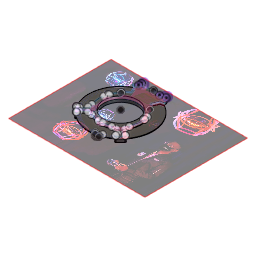
2023_02_18_DroneSoccerGoalFormat v3 (Autodesk Fusion 360 design; units mm, degrees)
Autodesk Fusion 360 part; units mm, degrees
note: some values were not read from the file. Set by a fixed rule: which face or edge a step refers to.
sketch "Sketch1" plane through (0, 0, 0) normal (0, 0, 1) x (1, 0, 0)
  circle A0 centre (0, 0) radius 30
  dimension "d1" = 60
  constraint coincident A0.centre origin
  measures "d1" diameter of A0
sketch "Sketch2" plane through (0, 0, 0) normal (0, 0, 1) x (1, 0, 0)
  line L0 (0.0532, -39.3057) -> (0.0532, -31.0517)
  line L1 (0.0532, -31.0517) -> (5.2469, -34.1533)
  line L2 (5.9386, -36.8958) -> (5.0815, -38.3311)
  line L3 (3.3644, -39.3057) -> (0.0532, -39.3057)
  line L4 (0.0532, -39.3057) -> (-3.258, -39.3057)
  line L5 (0.0532, -31.0517) -> (-5.1405, -34.1533)
  line L6 (-5.8322, -36.8958) -> (-4.9751, -38.3311)
  line L7 (-6.8576, -35.1787) -> (0.0532, -35.1787)
  line L8 (6.964, -35.1787) -> (0.0532, -35.1787)
  line L9 (0, 0) -> (-47, -35)
  line L10 (-47, -35) -> (-50.3407, -30.5139)
  line L11 (-50.6925, -28.9018) -> (-50.6943, -28.91)
  line L12 (-48.4045, -27.4507) -> (-45.0572, -29.2075)
  line L13 (-43.9952, -29.1241) -> (-35.2985, -22.6478)
  line L14 (-34.5132, -19.6138) -> (-37.2797, -13.4877)
  line L15 (-37.2164, -12.5462) -> (-35.0998, -9.1596)
  line L16 (-34.5983, -8.6155) -> (-32.5036, -7.0556)
  line L17 (-32.5036, -7.0556) -> (-24.2886, -18.0872)
  line L18 (0, 0) -> (0, 59)
  spline S0 degree 5 poles (0, 59) (-0.1827, 59.02) (-0.5488, 59.0563) (-1.1, 59.0994) (-1.8389, 59.134) (-2.7694, 59.1396) (-3.7076, 59.1081) (-4.6547, 59.0407) (-5.613, 58.9396) (-6.5861, 58.8081) (-7.5782, 58.6505) (-8.5938, 58.4709) (-9.637, 58.2733) (-10.7108, 58.0605) (-11.8165, 57.8337) (-12.953, 57.5917) (-14.1166, 57.3315) (-15.3013, 57.0494) (-16.4983, 56.7421) (-17.6962, 56.4075) (-18.8812, 56.0461) (-20.0369, 55.6616) (-21.1435, 55.2619) (-22.1835, 54.8583) (-23.1442, 54.4622) (-24.0258, 54.085) (-24.8384, 53.7327) (-25.6255, 53.4115) (-26.4188, 53.1074) (-27.16, 52.7706) (-27.7715, 52.3532) (-28.1746, 51.8252) (-28.3371, 51.2074) (-28.2837, 50.5744) (-28.0598, 50.0112) (-27.7047, 49.5822) (-27.218, 49.2903) (-26.5845, 49.0991) (-25.8011, 48.9581) (-24.9091, 48.8302) (-24.0064, 48.7073) (-23.2054, 48.5909) (-22.5994, 48.4787) (-22.2292, 48.3506) (-22.0395, 48.15) (-21.9198, 47.807) (-21.7816, 47.2816) (-21.5743, 46.5694) (-21.274, 45.6894) (-20.8803, 44.677) (-20.4088, 43.5748) (-19.8868, 42.4257) (-19.3496, 41.2728) (-18.8364, 40.1572) (-18.3867, 39.1164) (-18.0364, 38.183) (-17.8142, 37.3825) (-17.737, 36.733) (-17.8129, 36.2378) (-18.0462, 35.8787) (-18.443, 35.6058) (-19.0127, 35.3379) (-19.7561, 34.9915) (-20.657, 34.5019) (-21.6709, 33.8519) (-22.7199, 33.0863) (-23.7129, 32.2831) (-24.561, 31.5304) (-25.1962, 30.9002) (-25.5866, 30.4256) (-25.7572, 30.0716) (-25.7979, 29.7223) (-25.8113, 29.2507) (-25.8549, 28.5945) (-25.9293, 27.7723) (-26.0025, 26.8503) (-26.0238, 25.9241) (-25.9422, 25.0938) (-25.722, 24.4425) (-25.3404, 24.0341) (-24.7859, 23.9095) (-24.0562, 24.0833) (-23.1567, 24.5434) (-22.0989, 25.2573) (-20.899, 26.1767) (-19.5762, 27.2425) (-18.1514, 28.3898) (-16.6454, 29.5532) (-15.078, 30.6708) (-13.4656, 31.6909) (-11.8213, 32.5724) (-10.1553, 33.2835) (-8.4753, 33.8004) (-6.7868, 34.1063) (-5.0934, 34.19) (-3.3972, 34.045) (-2.0389, 33.7434) (-1.0197, 33.4125) (-0.3399, 33.1452) (0, 33) knots 0 0 0 0 0 0 0.01052632 0.02105263 0.03157895 0.04210526 0.05263158 0.06315789 0.07368421 0.08421053 0.09473684 0.10526316 0.11578947 0.12631579 0.13684211 0.14736842 0.15789474 0.16842105 0.17894737 0.18947368 0.2 0.21052632 0.22105263 0.23157895 0.24210526 0.25263158 0.26315789 0.27368421 0.28421053 0.29473684 0.30526316 0.31578947 0.32631579 0.33684211 0.34736842 0.35789474 0.36842105 0.37894737 0.38947368 0.4 0.41052632 0.42105263 0.43157895 0.44210526 0.45263158 0.46315789 0.47368421 0.48421053 0.49473684 0.50526316 0.51578947 0.52631579 0.53684211 0.54736842 0.55789474 0.56842105 0.57894737 0.58947368 0.6 0.61052632 0.62105263 0.63157895 0.64210526 0.65263158 0.66315789 0.67368421 0.68421053 0.69473684 0.70526316 0.71578947 0.72631579 0.73684211 0.74736842 0.75789474 0.76842105 0.77894737 0.78947368 0.8 0.81052632 0.82105263 0.83157895 0.84210526 0.85263158 0.86315789 0.87368421 0.88421053 0.89473684 0.90526316 0.91578947 0.92631579 0.93684211 0.94736842 0.95789474 0.96842105 0.97894737 0.98947368 1 1 1 1 1 1
  line L19 (-18.95, 56.1909) -> (-30.95, 51.1909)
  line L20 (-22.4748, 54.735) -> (-22.2313, 59.7077)
  line L21 (-21.5993, 60.1653) -> (-20.6365, 59.9004)
  line L22 (-20.1056, 61.8303) -> (-21.1577, 62.1197)
  arc A0 (-21.5993, 60.1653) -> (-22.2313, 59.7077) centre (-21.7319, 59.6832) ccw
  arc A1 (-21.3482, 62.5395) -> (-21.1577, 62.1197) centre (-21.0781, 62.409) ccw
  arc A2 (-20.6365, 59.9004) -> (-20.1056, 61.8303) centre (-18.7963, 60.4321) ccw
  spline S1 degree 5 poles (-21.3482, 62.5395) (-21.2588, 62.6491) (-21.0782, 62.8581) (-20.8015, 63.1417) (-20.4212, 63.4598) (-19.9273, 63.7557) (-19.4168, 63.9482) (-18.8942, 64.0357) (-18.3672, 64.0174) (-17.8475, 63.894) (-17.3471, 63.6688) (-16.8752, 63.348) (-16.4352, 62.9422) (-16.0208, 62.4678) (-15.6183, 61.9452) (-15.2114, 61.3961) (-14.786, 60.8402) (-14.334, 60.2934) (-13.8593, 59.7639) (-13.3785, 59.2517) (-12.9142, 58.7523) (-12.5748, 58.3573) (-12.3465, 58.0607) (-12.2072, 57.8625) (-12.1407, 57.7633) knots 0 0 0 0 0 0 0.05 0.1 0.15 0.2 0.25 0.3 0.35 0.4 0.45 0.5 0.55 0.6 0.65 0.7 0.75 0.8 0.85 0.9 0.95 1 1 1 1 1 1
  line L23 (-12.8077, 58.7587) -> (-11.4736, 56.7679)
  arc A3 (3.3644, -39.3057) -> (5.0815, -38.3311) centre (3.3644, -37.3057) ccw
  arc A4 (-4.9751, -38.3311) -> (-3.258, -39.3057) centre (-3.258, -37.3057) ccw
  arc A5 (5.9386, -36.8958) -> (5.2469, -34.1533) centre (4.2215, -35.8704) ccw
  arc A6 (-5.1405, -34.1533) -> (-5.8322, -36.8958) centre (-4.1151, -35.8704) ccw
  arc A7 (-49.0002, -27.3448) -> (-50.6943, -28.91) centre (-48.7383, -29.3275) ccw
  arc A8 (-50.6925, -28.9018) -> (-50.3407, -30.5139) centre (-48.7366, -29.3194) ccw
  arc A9 (-48.4045, -27.4507) -> (-49.0002, -27.3448) centre (-48.8693, -28.3361) ccw
  arc A10 (-45.0572, -29.2075) -> (-43.9952, -29.1241) centre (-44.5925, -28.3221) ccw
  arc A11 (-35.2985, -22.6478) -> (-34.5132, -19.6138) centre (-36.7917, -20.6427) ccw
  arc A12 (-37.2164, -12.5462) -> (-37.2797, -13.4877) centre (-36.3684, -13.0762) ccw
  arc A13 (-34.5983, -8.6155) -> (-35.0998, -9.1596) centre (-33.4038, -10.2196) ccw
  circle A14 centre (-18.7963, 60.4321) radius 1.9155
  spline S2 degree 5 poles (-22.2313, 59.7077) (-22.2233, 59.7803) (-22.2066, 59.9242) (-22.179, 60.136) (-22.1372, 60.4099) (-22.0758, 60.7375) (-22.0046, 61.0488) (-21.9225, 61.3423) (-21.8291, 61.617) (-21.7243, 61.8731) (-21.6092, 62.1121) (-21.5093, 62.2905) (-21.4303, 62.4176) (-21.3759, 62.4994) (-21.3482, 62.5395) knots 0 0 0 0 0 0 0.1 0.2 0.3 0.4 0.5 0.6 0.7 0.8 0.9 1 1 1 1 1 1
  point P0 (0.0532, -31.0517)
  point P1 (-5, 59)
  point P2 (-11, 58)
  point P3 (-19, 56)
  point P4 (-24.95, 53.6909)
  point P5 (-28, 52)
  point P6 (-28, 50)
  point P7 (-26, 49)
  point P8 (-22.554, 48.4463)
  point P9 (-22, 48)
  point P10 (-21, 45)
  point P11 (-18, 38)
  point P12 (-18, 36)
  point P13 (-20.4922, 34.5757)
  point P14 (-25.4906, 30.5144)
  point P15 (-25.803, 29.5)
  point P16 (-26, 26)
  point P17 (-25, 24)
  point P18 (-16, 30)
  point P19 (-19, 64)
  point P20 (-16.7409, 63.2086)
  point P21 (-14.5, 60.5)
  point P22 (-21.9, 61.4)
  dimension "d2" = 0.5
  dimension "d3" = 0.3
  dimension "d10" = 2
  dimension "d12" = 2
  dimension "d13" = 2
  dimension "d15" = 1
  dimension "d16" = 1
  dimension "d17" = 2.5
  dimension "d18" = 1
  dimension "d19" = 2
  constraint vertical L0
  constraint perpendicular L1 L2
  constraint perpendicular L0 L3
  constraint perpendicular L0 L4
  constraint midpoint L0 L7.end
  constraint perpendicular L0 L7
  constraint perpendicular L0 L8
  constraint equal L7 L8
  constraint coincident P0 L0.end
  constraint coincident L9.start L18.start
  constraint perpendicular L9 L10
  constraint parallel L9 L13
  constraint parallel L13 L16
  constraint coincident L9 L17.end
  constraint perpendicular L9 L17
  constraint vertical L18
  constraint coincident L18 S0.end
  constraint midpoint P4 L19
  constraint tangent L20 A0
  constraint tangent L21 A0
  constraint tangent L22 A1
  constraint tangent A1 S1
  constraint coincident S0 S1.end
  constraint midpoint S1.end L23
  constraint coincident S0 L20.start
  constraint tangent L2 A3
  constraint tangent L3 A3
  constraint tangent L4 A4
  constraint tangent L6 A4
  constraint equal A3 A4
  constraint coincident L8.start L2
  constraint coincident L8.start L1
  constraint tangent L2 A5
  constraint tangent L1 A5
  constraint equal A3 A5
  constraint coincident L7.start L6
  constraint coincident L7.start L5
  constraint tangent L6 A6
  constraint tangent L5 A6
  constraint equal A3 A6
  constraint tangent L11 A7
  constraint tangent L10 A8
  constraint tangent L11 A8
  constraint tangent A7 A9
  constraint tangent L12 A9
  constraint tangent L12 A10
  constraint tangent L13 A10
  constraint tangent L13 A11
  constraint tangent L14 A11
  constraint tangent L14 A12
  constraint tangent L15 A12
  constraint tangent L15 A13
  constraint tangent L16 A13
  constraint concentric A2 A14
  constraint coincident L22.start A14
  measures "d2" radius of A0
  measures "d3" radius of A1
  measures "d10" radius of A3
  measures "d12" radius of A7
  measures "d13" radius of A8
  measures "d15" radius of A9
  measures "d16" radius of A10
  measures "d17" radius of A11
  measures "d18" radius of A12
  measures "d19" radius of A13
extrude "Extrude1" add sketch "Sketch2" along normal blind 1 contours L18 S0 L19 | S0 L19 | S0 L19 makes body 1
extrude "Extrude12" add sketch "Sketch2" along normal blind 1 contours L21 L22 A0 A1 A14 S2 | S0 L20 L21 L22 A0 A1 A2 S1 A14 bodies 1
mirror "Mirror1" about plane through (0, 0, 0) normal (1, 0, 0) of bodies 1 merged
extrude "Extrude2" add sketch "Sketch2" along normal blind 1 separate body contours L0 L4 L6 L7 A4 A6 | L0 L2 L3 L8 A3 A5 | L0 L5 L7 A6 | L0 L1 L8 A5 makes body 2
extrude "Extrude4" add sketch "Sketch2" along normal blind 1 separate body contours L9 L10 L11 L12 L13 L14 L15 L16 L17 A7 A8 A9 A10 A11 A12 A13 makes body 3
mirror "Mirror2" about plane through (-24.2886, -18.0872, 0) normal (0.597266, -0.802043, 0) of bodies 3 merged
copy_body "CopyPasteBodies1" bodies 3 makes body 4
move_body "Move1" bodies 4 to x (-0.139173, 0.990268, 0) y (-0.990268, -0.139173, 0) z (0, 0, 1) at (0, 0, 0)
move_body "Move2" bodies 3 to x (0.992546, 0.121869, 0) y (-0.121869, 0.992546, 0) z (0, 0, 1) at (0, 0, 0)
copy_body "CopyPasteBodies2" bodies 2 makes body 5
move_body "Move3" bodies 5 to x (-0.258819, 0.965926, 0) y (-0.965926, -0.258819, 0) z (0, 0, 1) at (0, 0, 0)
copy_body "CopyPasteBodies3" bodies 2 makes body 6
move_body "Move4" bodies 6 to x (-0.258819, -0.965926, 0) y (0.965926, -0.258819, 0) z (0, 0, 1) at (0, 0, 0)
sketch "Sketch3" plane through (0, 0, 0) normal (0, 0, 1) x (1, 0, 0)
  circle A0 centre (0, 0) radius 30.1496
  circle A1 centre (0, 0) radius 37.2156
  circle A2 centre (0, 0) radius 57.7719
  constraint coincident A0.centre A1.centre
  constraint concentric A0 A1
  constraint concentric A1 A2
extrude "Extrude5" add sketch "Sketch3" along normal blind 1 contours A1 bodies 1 2 3 4 5 6
extrude "Extrude6" add 17 faces at (0.0566, -37.8765, 1) (-2.3425, -34.1233, 1) (34.115, -6.7759, 1) (23.5301, -22.5256, 1) (-22.9328, -23.1334, 1) (-32.3543, 11.0944, 1) (-20.4991, 28.1071, 1) (20.4991, 28.1071, 1) (33.5669, 6.5691, 1) (-32.2027, -32.0909, 1) (33.8058, -35.5758, 1) (-36.6005, 9.7484, 1) (-14.0329, 45.8265, 1) (14.0329, 45.8265, 1) (36.5712, 9.8579, 1) (-19.3015, 56.7106, 1) (19.3015, 56.7106, 1) along direction (0, 0, 1) blind 4 on bodies 1 bodies 1
sketch "Sketch4" plane through (0, 0, 5) normal (0, 0, 1) x (-1, 0, 0)
  arc A0 (-37.0215, -3.7963) -> (-37.1481, -3.9159) centre (-35.7132, -5.3091) ccw
  line L0 (-37.1481, -3.9159) -> (-38.3127, -5.1153)
  arc A1 (-38.3127, -5.1153) -> (-38.8096, -7.0261) centre (-36.8778, -6.5085) ccw
  line L1 (-38.8096, -7.0261) -> (-37.0956, -13.4228)
  arc A2 (-37.0956, -13.4228) -> (-35.7098, -14.8292) centre (-35.1638, -12.9052) ccw
  line L2 (-35.7098, -14.8292) -> (-34.1016, -15.2856)
  arc A3 (-34.1016, -15.2856) -> (-33.9117, -15.3296) centre (-33.5556, -13.3616) ccw
  arc A4 (-33.9117, -15.3296) -> (-25.9982, -26.6288) centre (0, 0) ccw
  spline S0 degree 5 poles (-25.9982, -26.6288) (-25.9968, -26.6728) (-25.9887, -26.8999) (-25.9656, -27.3118) (-25.918, -27.8971) (-25.8549, -28.5945) (-25.8113, -29.2507) (-25.7979, -29.7223) (-25.7572, -30.0716) (-25.5866, -30.4256) (-25.1962, -30.9002) (-24.561, -31.5304) (-23.7129, -32.2831) (-22.7199, -33.0863) (-21.6709, -33.8519) (-20.657, -34.5019) (-19.7561, -34.9915) (-19.0127, -35.3379) (-18.443, -35.6058) (-18.0462, -35.8787) (-17.8129, -36.2378) (-17.737, -36.733) (-17.8142, -37.3825) (-18.0364, -38.183) (-18.3867, -39.1164) (-18.8364, -40.1572) (-19.3496, -41.2728) (-19.8868, -42.4257) (-20.4088, -43.5748) (-20.8803, -44.677) (-21.274, -45.6894) (-21.5743, -46.5694) (-21.7816, -47.2816) (-21.9198, -47.807) (-22.0395, -48.15) (-22.2292, -48.3506) (-22.5994, -48.4787) (-23.2054, -48.5909) (-24.0064, -48.7073) (-24.9091, -48.8302) (-25.8011, -48.9581) (-26.5845, -49.0991) (-27.218, -49.2903) (-27.7047, -49.5822) (-28.0598, -50.0112) (-28.2837, -50.5744) (-28.3371, -51.2074) (-28.1746, -51.8252) (-27.7715, -52.3532) (-27.16, -52.7706) (-26.4188, -53.1074) (-25.6255, -53.4115) (-24.8384, -53.7327) (-24.077, -54.0628) (-23.4312, -54.3394) (-22.9326, -54.5479) (-22.6085, -54.6807) (-22.4748, -54.735) knots -0.770956 -0.770956 -0.770956 -0.770956 -0.770956 -0.770956 -0.768421 -0.757895 -0.747368 -0.736842 -0.726316 -0.715789 -0.705263 -0.694737 -0.684211 -0.673684 -0.663158 -0.652632 -0.642105 -0.631579 -0.621053 -0.610526 -0.6 -0.589474 -0.578947 -0.568421 -0.557895 -0.547368 -0.536842 -0.526316 -0.515789 -0.505263 -0.494737 -0.484211 -0.473684 -0.463158 -0.452632 -0.442105 -0.431579 -0.421053 -0.410526 -0.4 -0.389474 -0.378947 -0.368421 -0.357895 -0.347368 -0.336842 -0.326316 -0.315789 -0.305263 -0.294737 -0.284211 -0.273684 -0.263158 -0.252632 -0.242105 -0.231579 -0.224368 -0.224368 -0.224368 -0.224368 -0.224368 -0.224368
  spline S1 degree 5 poles (0, -59) (0.1827, -59.02) (0.5488, -59.0563) (1.1, -59.0994) (1.8389, -59.134) (2.7694, -59.1396) (3.7076, -59.1081) (4.6547, -59.0407) (5.613, -58.9396) (6.5861, -58.8081) (7.5782, -58.6505) (8.5938, -58.4709) (9.637, -58.2733) (10.5565, -58.0911) (11.2783, -57.9439) (11.7883, -57.8377) (12.0771, -57.7767) (12.1407, -57.7633) knots 0 0 0 0 0 0 0.010526 0.021053 0.031579 0.042105 0.052632 0.063158 0.073684 0.084211 0.094737 0.105263 0.115789 0.126316 0.129277 0.129277 0.129277 0.129277 0.129277 0.129277
  arc A5 (25.9982, -26.6288) -> (33.9597, -15.223) centre (0, 0) ccw
  arc A6 (33.9597, -15.223) -> (34.1292, -15.1828) centre (33.5831, -13.2588) ccw
  line L3 (34.1292, -15.1828) -> (35.7374, -14.7264)
  arc A7 (35.7374, -14.7264) -> (37.1232, -13.32) centre (35.1913, -12.8024) ccw
  line L4 (37.1232, -13.32) -> (38.8372, -6.9233)
  arc A8 (38.8372, -6.9233) -> (38.3402, -5.0125) centre (36.9053, -6.4057) ccw
  line L5 (38.3402, -5.0125) -> (37.1757, -3.8131)
  arc A9 (37.1757, -3.8131) -> (37.0332, -3.68) centre (35.7408, -5.2063) ccw
  arc A10 (37.0332, -3.68) -> (34.2626, 14.5283) centre (0, 0) ccw
  line L6 (34.2626, 14.5283) -> (35.41, 16.9882)
  arc A11 (35.41, 16.9882) -> (35.3581, 17.9305) centre (34.5037, 17.4109) ccw
  line L7 (35.3581, 17.9305) -> (31.8657, 23.6737)
  arc A12 (32.2753, 26.7808) -> (31.8657, 23.6737) centre (34.0017, 24.9726) ccw
  line L8 (32.2753, 26.7808) -> (40.118, 34.2687)
  arc A13 (41.1619, 34.4809) -> (40.118, 34.2687) centre (40.8085, 33.5454) ccw
  line L9 (41.1619, 34.4809) -> (44.6983, 33.1451)
  arc A14 (44.6983, 33.1451) -> (45.3025, 33.1125) centre (45.0517, 34.0806) ccw
  arc A15 (45.3025, 33.1125) -> (46.7928, 34.8684) centre (44.8009, 35.0486) ccw
  arc A16 (46.7928, 34.8684) -> (46.2467, 36.4215) centre (44.8002, 35.0404) ccw
  line L10 (46.2467, 36.4215) -> (38.5217, 44.5125)
  arc A17 (38.5217, 44.5125) -> (36.9956, 45.1298) centre (37.0752, 43.1314) ccw
  arc A18 (36.9956, 45.1298) -> (35.1727, 43.7223) centre (37.0835, 43.1317) ccw
  arc A19 (35.1727, 43.7223) -> (35.1773, 43.1173) centre (36.1281, 43.427) ccw
  line L11 (35.1773, 43.1173) -> (36.348, 39.5228)
  arc A20 (36.0878, 38.4899) -> (36.348, 39.5228) centre (35.3972, 39.2131) ccw
  line L12 (36.0878, 38.4899) -> (28.2451, 31.002)
  arc A21 (25.1224, 30.7365) -> (28.2451, 31.002) centre (26.5187, 32.8102) ccw
  line L13 (25.1224, 30.7365) -> (19.5468, 34.4909)
  arc A22 (19.5468, 34.4909) -> (18.608, 34.5862) centre (18.9883, 33.6614) ccw
  line L14 (18.608, 34.5862) -> (16.0977, 33.5539)
  arc A23 (16.0977, 33.5539) -> (5.9149, 36.7425) centre (0, 0) ccw
  arc A24 (5.9149, 36.7425) -> (5.8322, 36.8958) centre (4.1151, 35.8704) ccw
  line L15 (5.8322, 36.8958) -> (4.9751, 38.3311)
  arc A25 (4.9751, 38.3311) -> (3.258, 39.3057) centre (3.258, 37.3057) ccw
  line L16 (3.258, 39.3057) -> (-3.3644, 39.3057)
  arc A26 (-3.3644, 39.3057) -> (-5.0815, 38.3311) centre (-3.3644, 37.3057) ccw
  line L17 (-5.0815, 38.3311) -> (-5.9386, 36.8958)
  arc A27 (-5.9386, 36.8958) -> (-6.0303, 36.7238) centre (-4.2215, 35.8704) ccw
  arc A28 (-6.0303, 36.7238) -> (-15.1241, 34.0039) centre (0, 0) ccw
  line L18 (-15.1241, 34.0039) -> (-17.6036, 35.1081)
  arc A29 (-17.6036, 35.1081) -> (-18.5448, 35.0398) centre (-18.0104, 34.1946) ccw
  line L19 (-18.5448, 35.0398) -> (-24.2262, 31.4477)
  arc A30 (-27.34, 31.803) -> (-24.2262, 31.4477) centre (-25.5622, 33.5607) ccw
  line L20 (-27.34, 31.803) -> (-34.9636, 39.5138)
  arc A31 (-35.194, 40.5538) -> (-34.9636, 39.5138) centre (-34.2525, 40.2169) ccw
  line L21 (-35.194, 40.5538) -> (-33.9202, 44.1131)
  arc A32 (-33.9202, 44.1131) -> (-33.8981, 44.7177) centre (-34.8617, 44.45) ccw
  arc A33 (-33.8981, 44.7177) -> (-35.6797, 46.1771) centre (-35.8252, 44.1824) ccw
  arc A34 (-35.6797, 46.1771) -> (-37.223, 45.6041) centre (-35.8169, 44.1818) ccw
  line L22 (-37.223, 45.6041) -> (-45.178, 37.739)
  arc A35 (-45.178, 37.739) -> (-45.7686, 36.2023) centre (-43.7718, 36.3168) ccw
  arc A36 (-45.7686, 36.2023) -> (-44.3295, 34.4043) centre (-43.7723, 36.3251) ccw
  arc A37 (-44.3295, 34.4043) -> (-43.7246, 34.4194) centre (-44.0509, 35.3647) ccw
  line L23 (-43.7246, 34.4194) -> (-40.1512, 35.6527)
  arc A38 (-39.1138, 35.4105) -> (-40.1512, 35.6527) centre (-39.8249, 34.7075) ccw
  line L24 (-39.1138, 35.4105) -> (-31.4902, 27.6998)
  arc A39 (-31.1702, 24.5821) -> (-31.4902, 27.6998) centre (-33.268, 25.9421) ccw
  line L25 (-31.1702, 24.5821) -> (-34.8267, 18.9419)
  arc A40 (-34.8267, 18.9419) -> (-34.9057, 18.0015) centre (-33.9876, 18.3979) ccw
  line L26 (-34.9057, 18.0015) -> (-33.8297, 15.5096)
  arc A41 (-33.8297, 15.5096) -> (-37.0215, -3.7963) centre (0, 0) ccw
  circle A42 centre (0, 0) radius 30.1496
  line L27 (-37.1481, -3.9159) -> (-38.3127, -5.1153)
  arc A43 (-38.3127, -5.1153) -> (-38.8096, -7.0261) centre (-36.8778, -6.5085) ccw
  line L28 (-38.8096, -7.0261) -> (-37.0956, -13.4228)
  arc A44 (-37.0956, -13.4228) -> (-35.7098, -14.8292) centre (-35.1638, -12.9052) ccw
  line L29 (-35.7098, -14.8292) -> (-34.1016, -15.2856)
  arc A45 (-34.1016, -15.2856) -> (-33.9117, -15.3296) centre (-33.5556, -13.3616) ccw
  arc A46 (-33.9117, -15.3296) -> (-25.9982, -26.6288) centre (0, 0) ccw
  spline S2 degree 5 poles (-25.9982, -26.6288) (-25.9968, -26.6728) (-25.9887, -26.8999) (-25.9656, -27.3118) (-25.918, -27.8971) (-25.8549, -28.5945) (-25.8113, -29.2507) (-25.7979, -29.7223) (-25.7572, -30.0716) (-25.5866, -30.4256) (-25.1962, -30.9002) (-24.561, -31.5304) (-23.7129, -32.2831) (-22.7199, -33.0863) (-21.6709, -33.8519) (-20.657, -34.5019) (-19.7561, -34.9915) (-19.0127, -35.3379) (-18.443, -35.6058) (-18.0462, -35.8787) (-17.8129, -36.2378) (-17.737, -36.733) (-17.8142, -37.3825) (-18.0364, -38.183) (-18.3867, -39.1164) (-18.8364, -40.1572) (-19.3496, -41.2728) (-19.8868, -42.4257) (-20.4088, -43.5748) (-20.8803, -44.677) (-21.274, -45.6894) (-21.5743, -46.5694) (-21.7816, -47.2816) (-21.9198, -47.807) (-22.0395, -48.15) (-22.2292, -48.3506) (-22.5994, -48.4787) (-23.2054, -48.5909) (-24.0064, -48.7073) (-24.9091, -48.8302) (-25.8011, -48.9581) (-26.5845, -49.0991) (-27.218, -49.2903) (-27.7047, -49.5822) (-28.0598, -50.0112) (-28.2837, -50.5744) (-28.3371, -51.2074) (-28.1746, -51.8252) (-27.7715, -52.3532) (-27.16, -52.7706) (-26.4188, -53.1074) (-25.6255, -53.4115) (-24.8384, -53.7327) (-24.0258, -54.085) (-23.1442, -54.4622) (-22.1835, -54.8583) (-21.1435, -55.2619) (-20.0369, -55.6616) (-18.8812, -56.0461) (-17.6962, -56.4075) (-16.4983, -56.7421) (-15.3013, -57.0494) (-14.1166, -57.3315) (-12.953, -57.5917) (-11.8165, -57.8337) (-10.7108, -58.0605) (-9.637, -58.2733) (-8.5938, -58.4709) (-7.5782, -58.6505) (-6.5861, -58.8081) (-5.613, -58.9396) (-4.6547, -59.0407) (-3.7076, -59.1081) (-2.7694, -59.1396) (-1.8389, -59.134) (-1.1, -59.0994) (-0.5488, -59.0563) (-0.1827, -59.02) (0, -59) knots -0.77095641 -0.77095641 -0.77095641 -0.77095641 -0.77095641 -0.77095641 -0.76842105 -0.75789474 -0.74736842 -0.73684211 -0.72631579 -0.71578947 -0.70526316 -0.69473684 -0.68421053 -0.67368421 -0.66315789 -0.65263158 -0.64210526 -0.63157895 -0.62105263 -0.61052632 -0.6 -0.58947368 -0.57894737 -0.56842105 -0.55789474 -0.54736842 -0.53684211 -0.52631579 -0.51578947 -0.50526316 -0.49473684 -0.48421053 -0.47368421 -0.46315789 -0.45263158 -0.44210526 -0.43157895 -0.42105263 -0.41052632 -0.4 -0.38947368 -0.37894737 -0.36842105 -0.35789474 -0.34736842 -0.33684211 -0.32631579 -0.31578947 -0.30526316 -0.29473684 -0.28421053 -0.27368421 -0.26315789 -0.25263158 -0.24210526 -0.23157895 -0.22105263 -0.21052632 -0.2 -0.18947368 -0.17894737 -0.16842105 -0.15789474 -0.14736842 -0.13684211 -0.12631579 -0.11578947 -0.10526316 -0.09473684 -0.08421053 -0.07368421 -0.06315789 -0.05263158 -0.04210526 -0.03157895 -0.02105263 -0.01052632 0 0 0 0 0 0
  spline S3 degree 5 poles (0, -59) (0.1827, -59.02) (0.5488, -59.0563) (1.1, -59.0994) (1.8389, -59.134) (2.7694, -59.1396) (3.7076, -59.1081) (4.6547, -59.0407) (5.613, -58.9396) (6.5861, -58.8081) (7.5782, -58.6505) (8.5938, -58.4709) (9.637, -58.2733) (10.7108, -58.0605) (11.8165, -57.8337) (12.953, -57.5917) (14.1166, -57.3315) (15.3013, -57.0494) (16.4983, -56.7421) (17.6962, -56.4075) (18.8812, -56.0461) (20.0369, -55.6616) (21.1435, -55.2619) (22.1835, -54.8583) (23.1442, -54.4622) (24.0258, -54.085) (24.8384, -53.7327) (25.6255, -53.4115) (26.4188, -53.1074) (27.16, -52.7706) (27.7715, -52.3532) (28.1746, -51.8252) (28.3371, -51.2074) (28.2837, -50.5744) (28.0598, -50.0112) (27.7047, -49.5822) (27.218, -49.2903) (26.5845, -49.0991) (25.8011, -48.9581) (24.9091, -48.8302) (24.0064, -48.7073) (23.2054, -48.5909) (22.5994, -48.4787) (22.2292, -48.3506) (22.0395, -48.15) (21.9198, -47.807) (21.7816, -47.2816) (21.5743, -46.5694) (21.274, -45.6894) (20.8803, -44.677) (20.4088, -43.5748) (19.8868, -42.4257) (19.3496, -41.2728) (18.8364, -40.1572) (18.3867, -39.1164) (18.0364, -38.183) (17.8142, -37.3825) (17.737, -36.733) (17.8129, -36.2378) (18.0462, -35.8787) (18.443, -35.6058) (19.0127, -35.3379) (19.7561, -34.9915) (20.657, -34.5019) (21.6709, -33.8519) (22.7199, -33.0863) (23.7129, -32.2831) (24.561, -31.5304) (25.1962, -30.9002) (25.5866, -30.4256) (25.7572, -30.0716) (25.7979, -29.7223) (25.8113, -29.2507) (25.8549, -28.5945) (25.918, -27.8971) (25.9656, -27.3118) (25.9887, -26.8999) (25.9968, -26.6728) (25.9982, -26.6288) knots 0 0 0 0 0 0 0.01052632 0.02105263 0.03157895 0.04210526 0.05263158 0.06315789 0.07368421 0.08421053 0.09473684 0.10526316 0.11578947 0.12631579 0.13684211 0.14736842 0.15789474 0.16842105 0.17894737 0.18947368 0.2 0.21052632 0.22105263 0.23157895 0.24210526 0.25263158 0.26315789 0.27368421 0.28421053 0.29473684 0.30526316 0.31578947 0.32631579 0.33684211 0.34736842 0.35789474 0.36842105 0.37894737 0.38947368 0.4 0.41052632 0.42105263 0.43157895 0.44210526 0.45263158 0.46315789 0.47368421 0.48421053 0.49473684 0.50526316 0.51578947 0.52631579 0.53684211 0.54736842 0.55789474 0.56842105 0.57894737 0.58947368 0.6 0.61052632 0.62105263 0.63157895 0.64210526 0.65263158 0.66315789 0.67368421 0.68421053 0.69473684 0.70526316 0.71578947 0.72631579 0.73684211 0.74736842 0.75789474 0.76842105 0.77095641 0.77095641 0.77095641 0.77095641 0.77095641 0.77095641
  arc A47 (25.9982, -26.6288) -> (33.9597, -15.223) centre (0, 0) ccw
  arc A48 (33.9597, -15.223) -> (34.1292, -15.1828) centre (33.5831, -13.2588) ccw
  line L30 (34.1292, -15.1828) -> (35.7374, -14.7264)
  arc A49 (35.7374, -14.7264) -> (37.1232, -13.32) centre (35.1913, -12.8024) ccw
  line L31 (37.1232, -13.32) -> (38.8372, -6.9233)
  arc A50 (38.8372, -6.9233) -> (38.3402, -5.0125) centre (36.9053, -6.4057) ccw
  line L32 (38.3402, -5.0125) -> (37.1757, -3.8131)
  arc A51 (37.1757, -3.8131) -> (37.0332, -3.68) centre (35.7408, -5.2063) ccw
  arc A52 (37.0332, -3.68) -> (34.2626, 14.5283) centre (0, 0) ccw
  line L33 (34.2626, 14.5283) -> (35.41, 16.9882)
  arc A53 (35.41, 16.9882) -> (35.3581, 17.9305) centre (34.5037, 17.4109) ccw
  line L34 (35.3581, 17.9305) -> (31.8657, 23.6737)
  arc A54 (32.2753, 26.7808) -> (31.8657, 23.6737) centre (34.0017, 24.9726) ccw
  line L35 (32.2753, 26.7808) -> (40.118, 34.2687)
  arc A55 (41.1619, 34.4809) -> (40.118, 34.2687) centre (40.8085, 33.5454) ccw
  line L36 (41.1619, 34.4809) -> (44.6983, 33.1451)
  arc A56 (44.6983, 33.1451) -> (45.3025, 33.1125) centre (45.0517, 34.0806) ccw
  arc A57 (45.3025, 33.1125) -> (46.7928, 34.8684) centre (44.8009, 35.0486) ccw
  arc A58 (46.7928, 34.8684) -> (46.2467, 36.4215) centre (44.8002, 35.0404) ccw
  line L37 (46.2467, 36.4215) -> (38.5217, 44.5125)
  arc A59 (38.5217, 44.5125) -> (36.9956, 45.1298) centre (37.0752, 43.1314) ccw
  arc A60 (36.9956, 45.1298) -> (35.1727, 43.7223) centre (37.0835, 43.1317) ccw
  arc A61 (35.1727, 43.7223) -> (35.1773, 43.1173) centre (36.1281, 43.427) ccw
  line L38 (35.1773, 43.1173) -> (36.348, 39.5228)
  arc A62 (36.0878, 38.4899) -> (36.348, 39.5228) centre (35.3972, 39.2131) ccw
  line L39 (36.0878, 38.4899) -> (28.2451, 31.002)
  arc A63 (25.1224, 30.7365) -> (28.2451, 31.002) centre (26.5187, 32.8102) ccw
  line L40 (25.1224, 30.7365) -> (19.5468, 34.4909)
  arc A64 (19.5468, 34.4909) -> (18.608, 34.5862) centre (18.9883, 33.6614) ccw
  line L41 (18.608, 34.5862) -> (16.0977, 33.5539)
  arc A65 (16.0977, 33.5539) -> (5.9149, 36.7425) centre (0, 0) ccw
  arc A66 (5.9149, 36.7425) -> (5.8322, 36.8958) centre (4.1151, 35.8704) ccw
  line L42 (5.8322, 36.8958) -> (4.9751, 38.3311)
  arc A67 (4.9751, 38.3311) -> (3.258, 39.3057) centre (3.258, 37.3057) ccw
  line L43 (3.258, 39.3057) -> (-3.3644, 39.3057)
  arc A68 (-3.3644, 39.3057) -> (-5.0815, 38.3311) centre (-3.3644, 37.3057) ccw
  line L44 (-5.0815, 38.3311) -> (-5.9386, 36.8958)
  arc A69 (-5.9386, 36.8958) -> (-6.0303, 36.7238) centre (-4.2215, 35.8704) ccw
  arc A70 (-6.0303, 36.7238) -> (-15.1241, 34.0039) centre (0, 0) ccw
  line L45 (-15.1241, 34.0039) -> (-17.6036, 35.1081)
  arc A71 (-17.6036, 35.1081) -> (-18.5448, 35.0398) centre (-18.0104, 34.1946) ccw
  line L46 (-18.5448, 35.0398) -> (-24.2262, 31.4477)
  arc A72 (-27.34, 31.803) -> (-24.2262, 31.4477) centre (-25.5622, 33.5607) ccw
  line L47 (-27.34, 31.803) -> (-34.9636, 39.5138)
  arc A73 (-35.194, 40.5538) -> (-34.9636, 39.5138) centre (-34.2525, 40.2169) ccw
  line L48 (-35.194, 40.5538) -> (-33.9202, 44.1131)
  arc A74 (-33.9202, 44.1131) -> (-33.8981, 44.7177) centre (-34.8617, 44.45) ccw
  arc A75 (-33.8981, 44.7177) -> (-35.6797, 46.1771) centre (-35.8252, 44.1824) ccw
  arc A76 (-35.6797, 46.1771) -> (-37.223, 45.6041) centre (-35.8169, 44.1818) ccw
  line L49 (-37.223, 45.6041) -> (-45.178, 37.739)
  arc A77 (-45.178, 37.739) -> (-45.7686, 36.2023) centre (-43.7718, 36.3168) ccw
  arc A78 (-45.7686, 36.2023) -> (-44.3295, 34.4043) centre (-43.7723, 36.3251) ccw
  arc A79 (-44.3295, 34.4043) -> (-43.7246, 34.4194) centre (-44.0509, 35.3647) ccw
  line L50 (-43.7246, 34.4194) -> (-40.1512, 35.6527)
  arc A80 (-39.1138, 35.4105) -> (-40.1512, 35.6527) centre (-39.8249, 34.7075) ccw
  line L51 (-39.1138, 35.4105) -> (-31.4902, 27.6998)
  arc A81 (-31.1702, 24.5821) -> (-31.4902, 27.6998) centre (-33.268, 25.9421) ccw
  line L52 (-31.1702, 24.5821) -> (-34.8267, 18.9419)
  arc A82 (-34.8267, 18.9419) -> (-34.9057, 18.0015) centre (-33.9876, 18.3979) ccw
  line L53 (-34.9057, 18.0015) -> (-33.8297, 15.5096)
  arc A83 (-33.8297, 15.5096) -> (-37.0215, -3.7963) centre (0, 0) ccw
  arc A84 (-37.0215, -3.7963) -> (-37.1481, -3.9159) centre (-35.7132, -5.3091) ccw
  line L54 (-22.4748, -54.735) -> (-22.2313, -59.7077)
  spline S4 degree 5 poles (-22.2313, -59.7077) (-22.2233, -59.7803) (-22.2066, -59.9242) (-22.179, -60.136) (-22.1372, -60.4099) (-22.0758, -60.7375) (-22.0046, -61.0488) (-21.9225, -61.3423) (-21.8291, -61.617) (-21.7243, -61.8731) (-21.6092, -62.1121) (-21.5093, -62.2905) (-21.4303, -62.4176) (-21.3759, -62.4994) (-21.3482, -62.5395) knots 0 0 0 0 0 0 0.1 0.2 0.3 0.4 0.5 0.6 0.7 0.8 0.9 1 1 1 1 1 1
  spline S5 degree 5 poles (-21.3482, -62.5395) (-21.2588, -62.6491) (-21.0782, -62.8581) (-20.8015, -63.1417) (-20.4212, -63.4598) (-19.9273, -63.7557) (-19.4168, -63.9482) (-18.8942, -64.0357) (-18.3672, -64.0174) (-17.8475, -63.894) (-17.3471, -63.6688) (-16.8752, -63.348) (-16.4352, -62.9422) (-16.0208, -62.4678) (-15.6183, -61.9452) (-15.2114, -61.3961) (-14.786, -60.8402) (-14.334, -60.2934) (-13.8593, -59.7639) (-13.3785, -59.2517) (-12.9142, -58.7523) (-12.5748, -58.3573) (-12.3465, -58.0607) (-12.2072, -57.8625) (-12.1407, -57.7633) knots 0 0 0 0 0 0 0.05 0.1 0.15 0.2 0.25 0.3 0.35 0.4 0.45 0.5 0.55 0.6 0.65 0.7 0.75 0.8 0.85 0.9 0.95 1 1 1 1 1 1
  spline S6 degree 5 poles (-12.1407, -57.7633) (-12.0771, -57.7767) (-11.7883, -57.8377) (-11.2783, -57.9439) (-10.5565, -58.0911) (-9.637, -58.2733) (-8.5938, -58.4709) (-7.5782, -58.6505) (-6.5861, -58.8081) (-5.613, -58.9396) (-4.6547, -59.0407) (-3.7076, -59.1081) (-2.7694, -59.1396) (-1.8389, -59.134) (-1.1, -59.0994) (-0.5488, -59.0563) (-0.1827, -59.02) (0, -59) knots -0.129277 -0.129277 -0.129277 -0.129277 -0.129277 -0.129277 -0.126316 -0.115789 -0.105263 -0.094737 -0.084211 -0.073684 -0.063158 -0.052632 -0.042105 -0.031579 -0.021053 -0.010526 0 0 0 0 0 0
  spline S7 degree 5 poles (12.1407, -57.7633) (12.2072, -57.8625) (12.3465, -58.0607) (12.5748, -58.3573) (12.9142, -58.7523) (13.3785, -59.2517) (13.8593, -59.7639) (14.334, -60.2934) (14.786, -60.8402) (15.2114, -61.3961) (15.6183, -61.9452) (16.0208, -62.4678) (16.4352, -62.9422) (16.8752, -63.348) (17.3471, -63.6688) (17.8475, -63.894) (18.3672, -64.0174) (18.8942, -64.0357) (19.4168, -63.9482) (19.9273, -63.7557) (20.4212, -63.4598) (20.8015, -63.1417) (21.0782, -62.8581) (21.2588, -62.6491) (21.3482, -62.5395) knots -1 -1 -1 -1 -1 -1 -0.95 -0.9 -0.85 -0.8 -0.75 -0.7 -0.65 -0.6 -0.55 -0.5 -0.45 -0.4 -0.35 -0.3 -0.25 -0.2 -0.15 -0.1 -0.05 0 0 0 0 0 0
  spline S8 degree 5 poles (21.3482, -62.5395) (21.3759, -62.4994) (21.4303, -62.4176) (21.5093, -62.2905) (21.6092, -62.1121) (21.7243, -61.8731) (21.8291, -61.617) (21.9225, -61.3423) (22.0046, -61.0488) (22.0758, -60.7375) (22.1372, -60.4099) (22.179, -60.136) (22.2066, -59.9242) (22.2233, -59.7803) (22.2313, -59.7077) knots -1 -1 -1 -1 -1 -1 -0.9 -0.8 -0.7 -0.6 -0.5 -0.4 -0.3 -0.2 -0.1 0 0 0 0 0 0
  line L55 (22.2313, -59.7077) -> (22.4748, -54.735)
  spline S9 degree 5 poles (22.4748, -54.735) (22.6085, -54.6807) (22.9326, -54.5479) (23.4312, -54.3394) (24.077, -54.0628) (24.8384, -53.7327) (25.6255, -53.4115) (26.4188, -53.1074) (27.16, -52.7706) (27.7715, -52.3532) (28.1746, -51.8252) (28.3371, -51.2074) (28.2837, -50.5744) (28.0598, -50.0112) (27.7047, -49.5822) (27.218, -49.2903) (26.5845, -49.0991) (25.8011, -48.9581) (24.9091, -48.8302) (24.0064, -48.7073) (23.2054, -48.5909) (22.5994, -48.4787) (22.2292, -48.3506) (22.0395, -48.15) (21.9198, -47.807) (21.7816, -47.2816) (21.5743, -46.5694) (21.274, -45.6894) (20.8803, -44.677) (20.4088, -43.5748) (19.8868, -42.4257) (19.3496, -41.2728) (18.8364, -40.1572) (18.3867, -39.1164) (18.0364, -38.183) (17.8142, -37.3825) (17.737, -36.733) (17.8129, -36.2378) (18.0462, -35.8787) (18.443, -35.6058) (19.0127, -35.3379) (19.7561, -34.9915) (20.657, -34.5019) (21.6709, -33.8519) (22.7199, -33.0863) (23.7129, -32.2831) (24.561, -31.5304) (25.1962, -30.9002) (25.5866, -30.4256) (25.7572, -30.0716) (25.7979, -29.7223) (25.8113, -29.2507) (25.8549, -28.5945) (25.918, -27.8971) (25.9656, -27.3118) (25.9887, -26.8999) (25.9968, -26.6728) (25.9982, -26.6288) knots 0.224368 0.224368 0.224368 0.224368 0.224368 0.224368 0.231579 0.242105 0.252632 0.263158 0.273684 0.284211 0.294737 0.305263 0.315789 0.326316 0.336842 0.347368 0.357895 0.368421 0.378947 0.389474 0.4 0.410526 0.421053 0.431579 0.442105 0.452632 0.463158 0.473684 0.484211 0.494737 0.505263 0.515789 0.526316 0.536842 0.547368 0.557895 0.568421 0.578947 0.589474 0.6 0.610526 0.621053 0.631579 0.642105 0.652632 0.663158 0.673684 0.684211 0.694737 0.705263 0.715789 0.726316 0.736842 0.747368 0.757895 0.768421 0.770956 0.770956 0.770956 0.770956 0.770956 0.770956
  circle A85 centre (-18.7963, -60.4321) radius 1.9155
  circle A86 centre (18.7963, -60.4321) radius 1.9155
  spline S10 degree 5 poles (-21.3482, 62.5395) (-21.2588, 62.6491) (-21.0782, 62.8581) (-20.8015, 63.1417) (-20.4212, 63.4598) (-19.9273, 63.7557) (-19.4168, 63.9482) (-18.8942, 64.0357) (-18.3672, 64.0174) (-17.8475, 63.894) (-17.3471, 63.6688) (-16.8752, 63.348) (-16.4352, 62.9422) (-16.0208, 62.4678) (-15.6183, 61.9452) (-15.2114, 61.3961) (-14.786, 60.8402) (-14.334, 60.2934) (-13.8593, 59.7639) (-13.3785, 59.2517) (-12.9142, 58.7523) (-12.5748, 58.3573) (-12.3465, 58.0607) (-12.2072, 57.8625) (-12.1407, 57.7633) knots 0 0 0 0 0 0 0.05 0.1 0.15 0.2 0.25 0.3 0.35 0.4 0.45 0.5 0.55 0.6 0.65 0.7 0.75 0.8 0.85 0.9 0.95 1 1 1 1 1 1
  line L56 (-12.8077, 58.7587) -> (-11.4736, 56.7679)
  arc A87 (-20.6365, 59.9004) -> (-20.1056, 61.8303) centre (-18.7963, 60.4321) ccw
  line L57 (-22.4748, 54.735) -> (-22.2313, 59.7077)
  circle A88 centre (-18.7963, 60.4321) radius 1.9155
  spline S11 degree 5 poles (-22.2313, 59.7077) (-22.2233, 59.7803) (-22.2066, 59.9242) (-22.179, 60.136) (-22.1372, 60.4099) (-22.0758, 60.7375) (-22.0046, 61.0488) (-21.9225, 61.3423) (-21.8291, 61.617) (-21.7243, 61.8731) (-21.6092, 62.1121) (-21.5093, 62.2905) (-21.4303, 62.4176) (-21.3759, 62.4994) (-21.3482, 62.5395) knots 0 0 0 0 0 0 0.1 0.2 0.3 0.4 0.5 0.6 0.7 0.8 0.9 1 1 1 1 1 1
  point P0 (-19, 64)
  point P1 (-16.7409, 63.2086)
  point P2 (-14.5, 60.5)
  point P3 (-21.9, 61.4)
  constraint midpoint S10.end L56
  constraint concentric A87 A88
  constraint coincident A87.end A88
extrude "Extrude7" cut sketch "Sketch4" against normal blind 20 contours A0 L0 A1 L1 A2 L2 A3 A4 S0 S1 A5 A6 L3 A7 L4 A8 L5 A9 A10 L6 A11 L7 A12 L8 A13 L9 A14 A15 A16 L10 A17 A18 A19 L11 A20 L12 A21 L13 A22 L14 A23 A24 L15 A25 L16 A26 L17 A27 A28 L18 A29 L19 A30 L20 A31 L21 A32 A33 A34 L22 A35 A36 A37 L23 A38 L24 A39 L25 A40 L26 A41 L27 A43 L28 A44 L29 A45 A46 S2 S3 A47 A48 L30 A49 L31 A50 L32 A51 A52 L33 A53 L34 A54 L35 A55 L36 A56 A57 A58 L37 A59 A60 A61 L38 A62 L39 A63 L40 A64 L41 A65 A66 L42 A67 L43 A68 L44 A69 A70 L45 A71 L46 A72 L47 A73 L48 A74 A75 A76 L49 A77 A78 A79 L50 A80 L51 A81 L52 A82 L53 A83 A84 S6 S9 | S2 L54 S4 S5 | S3 S7 S8 L55 bodies 1
extrude "Extrude8" add sketch "Sketch4" against normal blind 5 contours A0 L0 A1 L1 A2 L2 A3 A4 S0 S1 A5 A6 L3 A7 L4 A8 L5 A9 A10 L6 A11 L7 A12 L8 A13 L9 A14 A15 A16 L10 A17 A18 A19 L11 A20 L12 A21 L13 A22 L14 A23 A24 L15 A25 L16 A26 L17 A27 A28 L18 A29 L19 A30 L20 A31 L21 A32 A33 A34 L22 A35 A36 A37 L23 A38 L24 A39 L25 A40 L26 A41 L27 A43 L28 A44 L29 A45 A46 S2 S3 A47 A48 L30 A49 L31 A50 L32 A51 A52 L33 A53 L34 A54 L35 A55 L36 A56 A57 A58 L37 A59 A60 A61 L38 A62 L39 A63 L40 A64 L41 A65 A66 L42 A67 L43 A68 L44 A69 A70 L45 A71 L46 A72 L47 A73 L48 A74 A75 A76 L49 A77 A78 A79 L50 A80 L51 A81 L52 A82 L53 A83 A84 S6 S9 | S2 L54 S4 S5 | S3 S7 S8 L55 bodies 1
move_body "Move5" bodies 1 to x (1, 0, 0) y (0, 1, 0) z (0, 0, 1) at (0, 0, -5)
extrude "Extrude9" add sketch "Sketch3" along normal blind 1 separate body contours A2 makes body 7
extrude "Extrude10" add sketch "Sketch4" along normal blind 5 separate body contours A0 L0 A1 L1 A2 L2 A3 A4 S0 S1 A5 A6 L3 A7 L4 A8 L5 A9 A10 L6 A11 L7 A12 L8 A13 L9 A14 A15 A16 L10 A17 A18 A19 L11 A20 L12 A21 L13 A22 L14 A23 A24 L15 A25 L16 A26 L17 A27 A28 L18 A29 L19 A30 L20 A31 L21 A32 A33 A34 L22 A35 A36 A37 L23 A38 L24 A39 L25 A40 L26 A41 L27 A43 L28 A44 L29 A45 A46 S2 S3 A47 A48 L30 A49 L31 A50 L32 A51 A52 L33 A53 L34 A54 L35 A55 L36 A56 A57 A58 L37 A59 A60 A61 L38 A62 L39 A63 L40 A64 L41 A65 A66 L42 A67 L43 A68 L44 A69 A70 L45 A71 L46 A72 L47 A73 L48 A74 A75 A76 L49 A77 A78 A79 L50 A80 L51 A81 L52 A82 L53 A83 A84 S6 S9 | S2 L54 S4 S5 | S3 S7 S8 L55 makes body 8
move_body "Move6" bodies 8 to x (1, 0, 0) y (0, 1, 0) z (0, 0, 1) at (0, 0, -5)
move_body "Move7" bodies 8 to x (1, 0, 0) y (0, 1, 0) z (0, 0, 1) at (0, 0, 1)
sketch "Sketch5" plane through (0, 0, 0) normal (0, 1, 0) x (1, 0, 0)
move_body "Move8" bodies 1 to x (1, 0, 0) y (0, 1, 0) z (0, 0, 1) at (0, 0, 0.5)
move_body "Move9" bodies 8 to x (1, 0, 0) y (0, 1, 0) z (0, 0, 1) at (0, 0, -0.5)
combine "Combine1" operation cut target body 8 tool bodies 7 keep tools
combine "Combine2" operation cut target body 1 tool bodies 7 keep tools
equation "d26 = 53 deg + 45 deg"
equation "d27 = 52 deg - 45 deg"
named bodies: "FrontPart", "GlassPart", "BackPart"
